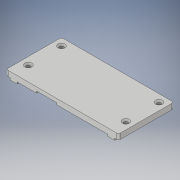
# Autodesk Inventor part: Link Adapter Top
Saved by Autodesk Inventor 2017 (Build 210142000, 142)
## iProperties
Created: 2020-09-10
Part Number: Link Adapter Top
Material: Generic
Document SubType Name: Modeling
Designer: Collin
Density: 1 g/cm^3
Appearance: Default
Author: Collin
Autodesk Inventor part; units mm, degrees
ref_plane "YZ Plane" through (0, 0, 0) normal (1, 0, 0) x (0, 1, 0)
ref_plane "XZ Plane" through (0, 0, 0) normal (0, 1, 0) x (-1, 0, 0)
ref_plane "XY Plane" through (0, 0, 0) normal (0, 0, 1) x (1, 0, 0)
sketch "Sketch1" plane through (0, 0, 0) normal (0, 1, 0) x (-1, 0, 0)
  line L0 (0, 0) -> (-61, 0)
  line L1 (-61, 0) -> (-61, -30)
  line L2 (-61, -30) -> (0, -30)
  line L3 (0, -30) -> (0, 0)
  dimension "d0" = 30
  dimension "d1" = 61
  constraints: 8 end point, 2 parallel, 1 horizontal, 1 perpendicular
  measures "d0" distance of L2.end L0.start
  measures "d1" distance of L1.end L2.end
extrude "Extrusion1" add sketch "Sketch1" along normal blind 3
fillet "Fillet1" radius 1 4 edges at (0, 1.5, 0) (61, 1.5, 0) (61, 1.5, -30) (0, 1.5, -30)
sketch "Sketch4" plane through (0, 0, 0) normal (0, -1, 0) x (1, 0, 0)
  line L0 (2.125, -2) -> (5.875, -2)
  line L1 (5.875, -2) -> (5.875, 0)
  line L2 (5.875, 0) -> (2.125, 0)
  line L3 (2.125, 0) -> (2.125, -2)
  line L4 (55.125, -2) -> (58.875, -2)
  line L5 (58.875, -2) -> (58.875, 0)
  line L6 (58.875, 0) -> (55.125, 0)
  line L7 (55.125, 0) -> (55.125, -2)
  line L8 (0, -29) -> (0, -1) projected
  line L9 (1, 0) -> (60, 0) projected
  line L10 (61, -1) -> (61, -29) projected
  point P0 (0, 0)
  dimension "d31" = 3.75
  dimension "d32" = 3.75
  dimension "d33" = 2
  dimension "d34" = 2
  dimension "d35" = 5.875
  dimension "d36" = 0
  dimension "d37" = 0
  dimension "d38" = 5.875
  constraints: 16 end point, 4 parallel, 2 horizontal, 2 perpendicular
  measures "d31" distance of L1.end L2.end
  measures "d32" distance of L5.end L6.end
  measures "d33" distance of L6.end L4.start
  measures "d34" distance of L2.end L0.start
  measures "d35" distance between parallel lines of L8 L1
  measures "d36" distance between parallel lines of L9 L2
  measures "d37" distance between parallel lines of L9 L6
  measures "d38" distance between parallel lines of L10 L7
extrude "Extrusion3" add sketch "Sketch4" along normal blind 1
sketch "Sketch2" plane through (0, 3, 0) normal (0, 1, 0) x (1, 0, 0)
  circle A0 centre (4, 8) radius 1
  line L0 (0, 0) -> (61, 0) projected
  line L1 (0, 30) -> (0, 0) projected
  circle A1 centre (57, 8) radius 1
  line L2 (61, 0) -> (61, 30) projected
  circle A2 centre (4, 26) radius 1
  circle A3 centre (57, 26) radius 1
  line L3 (61, 30) -> (0, 30) projected
  dimension "d4" = 8
  dimension "d5" = 4
  dimension "d6" = 2
  dimension "d7" = 2
  dimension "d8" = 4
  dimension "d9" = 8
  dimension "d10" = 2
  dimension "d11" = 2
  dimension "d12" = 4
  dimension "d13" = 4
  dimension "d14" = 4
  dimension "d15" = 4
  constraints: 4 centre point
  measures "d4" distance from line of L0 A0.centre
  measures "d5" distance from line of L1 A0.centre
  measures "d6" diameter of A0
  measures "d7" diameter of A1
  measures "d8" distance from line of L2 A1.centre
  measures "d9" distance from line of L0 A1.centre
  measures "d10" diameter of A2
  measures "d11" diameter of A3
  measures "d12" distance from line of L3 A2.centre
  measures "d13" distance from line of L1 A2.centre
  measures "d14" distance from line of L3 A3.centre
  measures "d15" distance from line of L2 A3.centre
hole "Hole1" at (4, 3, -26) at (4, 3, -8) at (57, 3, -8) at (57, 3, -26) direction (0, -1, 0) diameter 2.1 end through all countersink diameter 3.75 countersink angle 90
sketch "Sketch6" plane through (0, 0, 0) normal (0, -1, 0) x (1, 0, 0)
  line L0 (16.5, -10) -> (27.5, -10)
  line L1 (27.5, -10) -> (27.5, 0)
  line L2 (27.5, 0) -> (16.5, 0)
  line L3 (16.5, 0) -> (16.5, -10)
  line L4 (1, 0) -> (60, 0) projected
  line L5 (0, -29) -> (0, -1) projected
  line L6 (16.5, -30) -> (27.5, -30)
  line L7 (27.5, -30) -> (27.5, -20)
  line L8 (27.5, -20) -> (16.5, -20)
  line L9 (16.5, -20) -> (16.5, -30)
  line L10 (60, -30) -> (1, -30) projected
  point P0 (0, 0)
  dimension "d48" = 16.5
  dimension "d49" = 11
  dimension "d50" = 10
  dimension "d51" = 0
  dimension "d52" = 10
  dimension "d53" = 16.5
  dimension "d55" = 11
  dimension "d56" = 0
  constraints: 16 end point, 4 parallel, 2 horizontal, 2 perpendicular
  measures "d48" distance between parallel lines of L3 L5
  measures "d49" distance of L0.start L0.end
  measures "d50" distance of L2.end L0.start
  measures "d51" distance between parallel lines of L4 L2
  measures "d52" distance of L8.end L6.start
  measures "d53" distance between parallel lines of L5 L9
  measures "d55" distance of L6.start L6.end
  measures "d56" distance between parallel lines of L10 L6
extrude "Extrusion4" cut sketch "Sketch6" against normal blind 1
equation "\"d52\" = d50"
equation "\"d53\" = d48"
body "Solid1"
